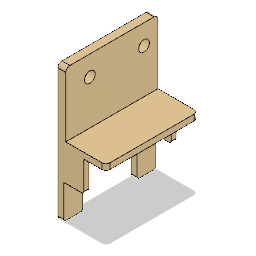
Mains_protector v5 (Autodesk Fusion 360 design; units mm, degrees)
Autodesk Fusion 360 part; units mm, degrees
sketch "Sketch1" plane through (0, 0, 0) normal (0, 0, 1) x (1, 0, 0)
  line L0 (4, 0) -> (4, 20)
  line L1 (4, 20) -> (0, 20)
  line L2 (0, 20) -> (0, 0)
  line L3 (0, 0) -> (4, 0)
  line L4 (4, 0) -> (4, -15)
  line L5 (4, -15) -> (0, -15)
  line L6 (0, -15) -> (0, 0)
  line L7 (0, -15) -> (3, -15)
  line L8 (3, -15) -> (3, -47)
  line L9 (3, -47) -> (0, -47)
  line L10 (0, -47) -> (0, -15)
  dimension "d1" = 20
  dimension "d2" = 4
  dimension "d3" = 15
  dimension "d4" = 32
  dimension "d5" = 3
  constraint vertical L0
  constraint horizontal L1
  constraint vertical L2
  constraint coincident L2.end L3.start
  constraint horizontal L3
  constraint vertical L4
  constraint horizontal L5
  constraint vertical L6
  constraint collinear L0 L4
  constraint horizontal L7
  constraint vertical L8
  constraint horizontal L9
  constraint vertical L10
  constraint coincident L0.start L3.end
  measures "d1" distance of L0.start L0.end
  measures "d2" distance of L0.end L1.end
  measures "d3" distance of L0.start L4.end
  measures "d4" distance of L7.end L8.end
  measures "d5" distance of L8.end L9.end
extrude "Extrude1" add sketch "Sketch1" along normal blind 46
sketch "Sketch2" plane through (4, 0, 0) normal (1, 0, 0) x (0, 0, -1)
  line L0 (0, -15) -> (0, 20)
  line L1 (0, 20) -> (-46, 20)
  line L2 (-46, 20) -> (-46, -15)
  line L3 (-46, -15) -> (0, -15)
  line L4 (-46, 10) -> (0, 10) construction
  circle A0 centre (-34, 10) radius 2.7
  circle A1 centre (-7, 10) radius 2.7
  line L5 (-46, -12) -> (0, -12)
  line L6 (0, -47) -> (0, -15) construction
  line L7 (0, -15) -> (-46, -15) construction
  line L8 (-46, -15) -> (-46, -47) construction
  line L9 (-46, -47) -> (0, -47) construction
  line L10 (-23, 20) -> (-23, -47) construction
  line L11 (-36.5, -25) -> (-9.5, -25)
  line L12 (-9.5, -25) -> (-9.5, -47)
  line L13 (-9.5, -47) -> (-36.5, -47)
  line L14 (-36.5, -47) -> (-36.5, -25)
  dimension "d8" = 5.4
  dimension "d9" = 5.4
  dimension "d10" = 3
  dimension "d11" = 27
  dimension "d12" = 22
  dimension "d17" = 7
  dimension "d18" = 12
  dimension "d19" = 11.5
  dimension "d24" = 25
  dimension "d25" = 15
  constraint coincident L2 L4.start
  constraint coincident L0 L4.end
  constraint perpendicular L0 L4
  constraint coincident L4 A0.centre
  constraint coincident L4 A1.centre
  constraint coincident L2 L5.start
  constraint coincident L0 L5.end
  constraint perpendicular L0 L5
  constraint midpoint L1 L10.start
  constraint midpoint L9 L10.end
  constraint horizontal L11
  constraint vertical L12
  constraint horizontal L13
  constraint vertical L14
  constraint midpoint L10.end L13
  measures "d8" diameter of A1
  measures "d9" diameter of A0
  measures "d10" distance of L3 L5
  measures "d11" distance of L12 L14
  measures "d12" distance of L11.end L12.end
  measures "d17" distance of L0 A1.centre
  measures "d18" distance of L2 A0.centre
  measures "d19" distance of L6 L12
  measures "d24" distance of L3 A1.centre
extrude "Extrude3" add sketch "Sketch2" along normal blind 20 contours L0 L2 L3 L5
extrude "Extrude2" cut sketch "Sketch2" against normal through all contours A0 | A1 | L11 L12 L13 L14
sketch "Sketch3" plane through (3, 0, 0) normal (1, 0, 0) x (0, 0, -1)
  line L0 (-9.5, -25) -> (-9.5, -47)
  line L1 (-9.5, -47) -> (0, -47)
  line L2 (0, -47) -> (0, -15)
  line L3 (0, -15) -> (-46, -15)
  line L4 (-46, -15) -> (-46, -47)
  line L5 (-46, -47) -> (-36.5, -47)
  line L6 (-36.5, -47) -> (-36.5, -25)
  line L7 (-36.5, -25) -> (-9.5, -25)
  line L8 (-46, -15) -> (-43.5, -15)
  line L9 (-43.5, -15) -> (-43.5, -30)
  line L10 (-43.5, -30) -> (-46, -30)
  line L11 (-46, -30) -> (-46, -15)
  line L12 (0, -15) -> (-2.5, -15)
  line L13 (-2.5, -15) -> (-2.5, -30)
  line L14 (-2.5, -30) -> (0, -30)
  line L15 (0, -30) -> (0, -15)
  dimension "d26" = 15
  dimension "d27" = 2.5
  dimension "d28" = 2.5
  constraint horizontal L8
  constraint vertical L9
  constraint horizontal L10
  constraint vertical L11
  constraint coincident L3.end L4.start
  constraint horizontal L12
  constraint vertical L13
  constraint horizontal L14
  constraint vertical L15
  constraint coincident L2.end L3.start
  constraint collinear L10 L14
  measures "d26" distance of L3.end L10.end
  measures "d27" distance of L9.end L10.end
  measures "d28" distance of L13.end L14.end
extrude "Extrude4" add sketch "Sketch3" along normal blind 10 contours L2 L3 L12 L13 L14 L15 | L3 L4 L8 L9 L10 L11
fillet "Fillet1" radius 2 4 edges at (2, 20, 46) (2, 20, 0) (24, -13.5, 0) (24, -13.5, 46)
fillet "Fillet2" radius 1 8 edges at (1.5, -25, 36.5) (1.5, -25, 9.5) (1.5, -47, 9.5) (1.5, -47, 0) (1.5, -47, 36.5) (1.5, -47, 46) (13, -30, 44.75) (13, -30, 1.25)
equation "d9 = d8"
equation "d28 = d27"
